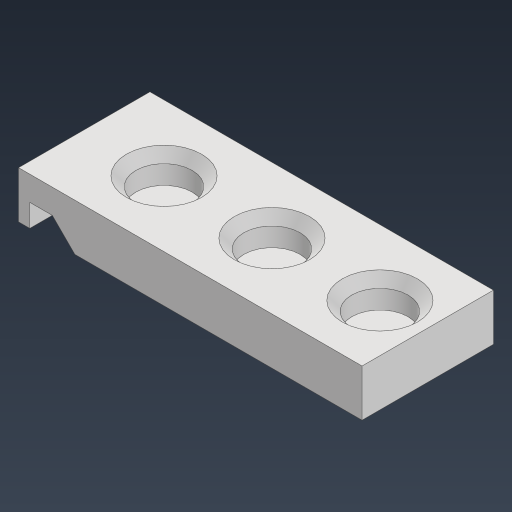
# Autodesk Inventor part: glue_test_flex_2
Saved by Autodesk Inventor 2023 (Build 270158000, 158)
## iProperties
Created: 2025-12-21
Part Number: glue_test_flex_2
Material: Generic
Document SubType Name: Modeling
Designer: szymo
Density: 1 g/cm^3
Appearance: Default
Author: szymo
Autodesk Inventor part; units mm, degrees
ref_plane "YZ Plane" through (0, 0, 0) normal (1, 0, 0) x (0, 1, 0)
ref_plane "XZ Plane" through (0, 0, 0) normal (0, 1, 0) x (-1, 0, 0)
ref_plane "XY Plane" through (0, 0, 0) normal (0, 0, 1) x (1, 0, 0)
sketch "Sketch1" plane through (0, 0, 0) normal (0, 1, 0) x (-1, 0, 0)
  line L0 (-10, 3.5) -> (10, 3.5)
  line L1 (10, 3.5) -> (10, -3.5)
  line L2 (10, -3.5) -> (-10, -3.5)
  line L3 (-10, -3.5) -> (-10, 3.5)
  line L4 (-10, 3.5) -> (10, -3.5) construction
  line L5 (10, 3.5) -> (-10, -3.5) construction
  line L6 (-10, 0) -> (10, 0) construction
  circle A0 centre (-5.75, 0) radius 1.5
  circle A1 centre (5.75, 0) radius 1.5
  circle A2 centre (0, 0) radius 1.5
  line L7 (-8.3, 3.5) -> (-8.3, -3.5)
  point P0 (0, 0)
  dimension "d0" = 7
  dimension "d1" = 20
  dimension "d2" = 3
  dimension "d3" = 3
  dimension "d4" = 3
  dimension "d5" = 5.75
  dimension "d6" = 5.75
  dimension "d7" = 4.25
  dimension "d8" = 4.25
  dimension "d16" = 1.7
  constraints: 16 end point, 5 midpoint, 4 point on line, 3 centre point, 2 parallel, 2 perpendicular, 1 horizontal
  measures "d0" distance of L0.end L1.end
  measures "d1" distance of L1.end L2.end
  measures "d2" diameter of A0
  measures "d3" diameter of A1
  measures "d4" diameter of A2
  measures "d5" distance of A2.centre A0.centre
  measures "d6" distance of A1.centre A2.centre
  measures "d7" distance from line of L1 A1.centre
  measures "d8" distance from line of L3 A0.centre
  measures "d16" distance between parallel lines of L3 L7
extrude "Extrusion1" add sketch "Sketch1" along normal blind 2.5 contours L0 L1 L2 L7
extrude "Extrusion2" add sketch "Sketch1" along normal blind 1 contours A0 | A1 | A2
chamfer "Chamfer1" distance 0.5 angle 45 3 edges at (7.25, 2.5, 0) (1.5, 2.5, 0) (-4.25, 2.5, 0)
sketch "Sketch2" plane through (-10, 0, 3.5) normal (0, 0, 1) x (1, 0, 0)
  line L0 (0, 0) -> (18.3, 0) projected
  line L1 (18.3, 0) -> (18.3, 2.5) projected
  line L2 (0, 2.5) -> (18.3, 2.5) projected
  line L3 (0, 0) -> (0, 2.5) projected
  line L4 (2.75, 2) -> (5.75, 2) projected
  line L5 (6.25, 2.5) -> (2.25, 2.5) projected
  line L6 (2.75, 2) -> (2.25, 2.5)
  line L7 (3, 0) -> (1.8, 1.2)
  line L8 (0.6, 1.2) -> (0.6, 0)
  line L9 (2.75, 1) -> (5.75, 1) projected
  line L10 (2.75, 2) -> (2.75, 1)
  line L11 (2.75, 2) -> (2.75, 1) projected
  line L12 (5.75, 1) -> (5.75, 2)
  line L13 (5.75, 2) -> (6.25, 2.5)
  line L14 (1.8, 1.2) -> (0.6, 1.2)
  point P0 (10, 0)
  dimension "d17" = 0.6
  dimension "d18" = 90
  dimension "d19" = 45
  dimension "d21" = 1.2
  dimension "d22" = 1.2
  dimension "d23" = 0.5303
  constraints: 15 end point, 2 equal length, 2 point on line, 1 perpendicular
  measures "d17" distance of L0.start L8.end
  measures "d18" angle of L0 L8
  measures "d19" angle of L0 L7
  measures "d21" distance of L7.end L8.start
  measures "d22" distance of L8.start L8.end
  measures "d23" distance from line of L7 L9.start
extrude "Extrusion3" cut sketch "Sketch2" against normal through all contours L8 L14 L7 L0
equation "\"d6\" = d5"
equation "\"d7\" = d5 - 0.5 * d3"
equation "\"d8\" = d5 - 0.5 * d2"
equation "\"d21\" = d22"
body "Solid1"
